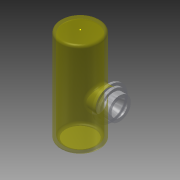
# Autodesk Inventor part: X-Ray Tube
Saved by Autodesk Inventor 2015 SP1 (Build 190203100, 203)
## iProperties
Created: 2015-03-02
Part Number: X-Ray Tube
Material: Glass
Document SubType Name: Modeling
Designer: pltwe4
Density: 2.18 g/cm^3
Appearance: Clear - Yellow
Author: pltwe4
Autodesk Inventor part; units mm, degrees
ref_plane "XZ Plane" through (0, 0, 0) normal (0, 1, 0) x (-1, 0, 0)
ref_plane "XY Plane" through (0, 0, 0) normal (0, 0, 1) x (1, 0, 0)
sketch "Sketch1" plane through (0, 0, 0) normal (0, 0, 1) x (1, 0, 0)
  circle A0 centre (0, 0) radius 14.925
  dimension "d0" = 29.85
  constraints: 1 centre point, 1 coincident
  measures "d0" diameter of A0
extrude "Extrusion1" add sketch "Sketch1" along normal mid plane 71.7
ref_plane "Work Plane1" through (14.925, 0, 0) normal (1, 0, 0) x (0, 1, 0)
sketch "Sketch2" plane through (14.925, 0, 0) normal (1, 0, 0) x (0, 1, 0)
  line L0 (-14.925, -35.85) -> (14.925, -35.85) projected
  line L1 (14.925, 35.85) -> (-14.925, 35.85) projected
  circle A0 centre (0, -1.03) radius 8.575
  line L2 (0, 50.19) -> (0, -50.19) projected
  point P0 (0, 0)
  dimension "d3" = 34.82
  dimension "d4" = 17.15
  constraints: 1 centre point, 1 point on line
  measures "d3" distance from line of L0 A0.centre
  measures "d4" diameter of A0
extrude "Extrusion2" add sketch "Sketch2" against normal up to surface round surface about axis through (0, 0, 0) along (0, 0, 1) radius 14.925 far side no
extrude "Extrusion3" add sketch "Sketch2" along normal blind 5.33
sketch "Sketch3" plane through (20.255, 0, -1.03) normal (1, 0, 0) x (0, 0, -1)
  circle A0 centre (0, 0) radius 8.575 projected
  circle A1 centre (0, 0) radius 12.575
  point P0 (-1.03, 0)
  dimension "d9" = 4
  constraints: 1 centre point, 1 coincident
  measures "d9" radial gap between concentric circles of A0 A1
fillet "Fillet1" radius 2 5 edges at (13.6017, 6.1441, 4.9517) (12.2267, 8.5595, -0.514) (13.4268, 6.5174, -6.6026) (13.2583, -6.8537, -6.1833) (13.6009, -6.1459, 4.9499)
extrude "Extrusion8" add sketch "Sketch3" along normal blind 3 contours A0 | A1
sketch "Sketch6" plane through (23.255, 0, -1.03) normal (1, 0, 0) x (0, 0, -1)
  circle A0 centre (0, 0) radius 12.575 projected
  circle A1 centre (0, 0) radius 10.575
  point P0 (-1.03, 0)
  dimension "d22" = 2
  constraints: 1 centre point, 1 coincident
  measures "d22" radial gap between concentric circles of A0 A1
extrude "Extrusion9" add sketch "Sketch6" along normal blind 2 contours A1
sketch "Sketch7" plane through (25.255, 0, -1.03) normal (1, 0, 0) x (0, 0, -1)
  circle A0 centre (0, 0) radius 8.575 projected
  point P0 (-1.03, 0)
extrude "Extrusion10" add sketch "Sketch7" along normal blind 4.44
fillet "Fillet2" radius 2 1 edges at (20.255, 0, 11.545)
sketch "Sketch8" plane through (0, 0, 0) normal (0, 1, 0) x (-1, 0, 0)
  line L0 (-29.695, 7.545) -> (-29.695, -9.605) projected
  line L1 (-25.255, -9.605) -> (-25.255, 7.545) projected
  line L2 (-29.695, 7.545) -> (-29.695, -9.605) projected
  line L3 (-29.695, 5.0115) -> (0, -1.03)
  line L4 (0, -1.03) -> (-29.695, -7.0715)
  line L5 (-29.695, -1.03) -> (-7.1474, -1.03) construction
  line L6 (0, -18.696) -> (0, 44.941) projected
  line L7 (0, -1.03) -> (-29.695, -1.03)
  line L8 (-29.695, -1.03) -> (-29.695, -7.0715)
  point P0 (0, 0)
  dimension "d28" = 23
  constraints: 10 end point, 3 point on line, 2 collinear, 1 midpoint, 1 perpendicular, 1 other
  measures "d28" angle of L4 L3
revolve "Revolution1" cut sketch "Sketch8" angle 360 about axis through (29.695, 0, -1.03) along (-1, 0, 0) contours L7 L1 L4 L0 | L7 L4 L1
sketch "Sketch9" plane through (0, 0, 35.85) normal (0, 0, 1) x (1, 0, 0)
  point P0 (0, 0)
sketch "Sketch10" plane through (0, 0, 35.85) normal (0, 0, 1) x (1, 0, 0)
  circle A0 centre (0, 0) radius 12.925
  circle A1 centre (0, 0) radius 14.925 projected
  dimension "d31" = 2
  constraints: 1 centre point, 1 coincident
  measures "d31" radial gap between concentric circles of A1 A0
extrude "Extrusion11" cut sketch "Sketch10" against normal blind 70.7 contours A0
fillet "Fillet3" radius 2 1 edges at (-12.925, 0, -34.85)
fillet "Fillet4" radius 2 1 edges at (-14.925, 0, -35.85)
fillet "Fillet5" radius 2 3 edges at (12.6655, -2.5768, -1.03) (12.7754, 1.9609, -2.736) (12.7754, 1.9609, 0.676)
sketch "Sketch11" plane through (0, 0, 35.85) normal (0, 0, 1) x (1, 0, 0)
  circle A0 centre (0, 0) radius 12.925 projected
extrude "Extrusion12" add sketch "Sketch11" against normal blind 1
fillet "Fillet6" radius 2 1 edges at (-12.925, 0, 34.85)
fillet "Fillet7" radius 2 1 edges at (-14.925, 0, 35.85)
body "Solid1"
